Autodesk Fusion 360 part; units mm, degrees
note: some values were not read from the file. Chosen so that the rebuilt part matches the saved one: which bodies a step acts on.
(part 2 of 3)
extrude "Extrude1'''''''''''''''''''''''" add sketch "FingerTech_Mini_Switch_Envelope_Outline" along normal blind 6.35 from surface at 49 separate body makes body 27 in component "FingerTech_Mini_Switch_Envelope"
sketch "FingerTech_Mount_Holes_M2" plane through (0, 0, 0) normal (0, 0, 1) x (1, 0, 0) in component "FingerTech_Mini_Switch_Envelope"
  circle A0 centre (38.19, -70) radius 1
  circle A1 centre (45.81, -70) radius 1
extrude "Extrude2''''''''''''''''" cut sketch "FingerTech_Mount_Holes_M2" along normal blind 9 from surface at 48 bodies 27 in component "FingerTech_Mini_Switch_Envelope"
sketch "FingerTech_Access_Patch" plane through (0, 0, 0) normal (0, 0, 1) x (1, 0, 0) in component "Top_Cover"
  line L0 (31, -79) -> (53, -79)
  line L1 (53, -79) -> (53, -61)
  line L2 (53, -61) -> (31, -61)
  line L3 (31, -61) -> (31, -79)
extrude "Extrude7''''" add sketch "FingerTech_Access_Patch" along normal blind 2 from surface at 83 bodies 6 in component "Top_Cover"
sketch "FingerTech_Hex_Access_6mm" plane through (0, 0, 0) normal (0, 0, 1) x (1, 0, 0) in component "Top_Cover"
  circle A0 centre (42, -70) radius 3
extrude "Extrude8''" cut sketch "FingerTech_Hex_Access_6mm" along normal blind 4 from surface at 82 bodies 6 in component "Top_Cover"
sketch "Lifter_Spatula_62mm_Side_Profile" plane through (0, 0, 0) normal (1, 0, 0) x (0, 0, -1) in component "Lifter_Spatula_62mm"
  line L0 (-27, 70) -> (-5.8, 112)
  line L1 (-5.8, 112) -> (-8.5, 112)
  line L2 (-8.5, 112) -> (-30, 72)
  line L3 (-30, 72) -> (-27, 70)
extrude "Extrude1''''''''''''''''''''''''" add sketch "Lifter_Spatula_62mm_Side_Profile" along normal blind 62 from surface at -31 separate body makes body 28 in component "Lifter_Spatula_62mm"
sketch "Lifter_Hinge_Boss_Outline" plane through (0, 0, 0) normal (0, 0, 1) x (1, 0, 0) in component "Lifter_Hinge_Boss"
  line L0 (-30, 64) -> (30, 64)
  line L1 (30, 64) -> (30, 74)
  line L2 (30, 74) -> (-30, 74)
  line L3 (-30, 74) -> (-30, 64)
extrude "Extrude1'''''''''''''''''''''''''" add sketch "Lifter_Hinge_Boss_Outline" along normal blind 9 from surface at 27 separate body makes body 29 in component "Lifter_Hinge_Boss"
sketch "Hinge_Clearance_Bore_6p4mm" plane through (0, 0, 0) normal (1, 0, 0) x (0, 0, -1) in component "Lifter_Hinge_Boss"
  circle A0 centre (-31.5, 68) radius 3.2
extrude "Extrude2'''''''''''''''''" cut sketch "Hinge_Clearance_Bore_6p4mm" along normal mid plane 100 bodies 29 in component "Lifter_Hinge_Boss"
sketch "Lifter_Pivot_Support_L_Outline" plane through (0, 0, 0) normal (0, 0, 1) x (1, 0, 0) in component "Lifter_Pivot_Support_L"
  line L0 (-35, 61) -> (-32, 61)
  line L1 (-32, 61) -> (-32, 76)
  line L2 (-32, 76) -> (-35, 76)
  line L3 (-35, 76) -> (-35, 61)
extrude "Extrude1''''''''''''''''''''''''''" add sketch "Lifter_Pivot_Support_L_Outline" along normal blind 17 from surface at 24 separate body makes body 30 in component "Lifter_Pivot_Support_L"
sketch "Lifter_Pivot_Support_R_Outline" plane through (0, 0, 0) normal (0, 0, 1) x (1, 0, 0) in component "Lifter_Pivot_Support_R"
  line L0 (32, 61) -> (35, 61)
  line L1 (35, 61) -> (35, 76)
  line L2 (35, 76) -> (32, 76)
  line L3 (32, 76) -> (32, 61)
extrude "Extrude1'''''''''''''''''''''''''''" add sketch "Lifter_Pivot_Support_R_Outline" along normal blind 17 from surface at 24 separate body makes body 31 in component "Lifter_Pivot_Support_R"
sketch "Left_Pivot_Bore_6p4mm" plane through (0, 0, 0) normal (1, 0, 0) x (0, 0, -1) in component "Lifter_Pivot_Support_L"
  circle A0 centre (-31.5, 68) radius 3.2
extrude "Extrude2''''''''''''''''''" cut sketch "Left_Pivot_Bore_6p4mm" along normal mid plane 100 bodies 30 in component "Lifter_Pivot_Support_L"
sketch "Right_Pivot_Bore_6p4mm" plane through (0, 0, 0) normal (1, 0, 0) x (0, 0, -1) in component "Lifter_Pivot_Support_R"
  circle A0 centre (-31.5, 68) radius 3.2
extrude "Extrude2'''''''''''''''''''" cut sketch "Right_Pivot_Bore_6p4mm" along normal mid plane 100 bodies 31 in component "Lifter_Pivot_Support_R"
sketch "Lifter_Pivot_Pin_6mm_Section" plane through (0, 0, 0) normal (1, 0, 0) x (0, 0, -1) in component "Lifter_Pivot_Pin_6mm"
  circle A0 centre (-31.5, 68) radius 3
extrude "Extrude1''''''''''''''''''''''''''''" add sketch "Lifter_Pivot_Pin_6mm_Section" along normal blind 72 from surface at -36 separate body makes body 32 in component "Lifter_Pivot_Pin_6mm"
sketch "Pin_End_Trim_L" plane through (0, 0, 0) normal (1, 0, 0) x (0, 0, -1) in component "Lifter_Pivot_Pin_6mm"
  circle A0 centre (-31.5, 68) radius 3.5
extrude "Extrude2''''''''''''''''''''" cut sketch "Pin_End_Trim_L" along normal blind 1.3 from surface at -36.1 bodies 32 in component "Lifter_Pivot_Pin_6mm"
sketch "Pin_End_Trim_R" plane through (0, 0, 0) normal (1, 0, 0) x (0, 0, -1) in component "Lifter_Pivot_Pin_6mm"
  circle A0 centre (-31.5, 68) radius 3.5
extrude "Extrude3''''''''''''''''" cut sketch "Pin_End_Trim_R" along normal blind 1.3 from surface at 34.8 bodies 32 in component "Lifter_Pivot_Pin_6mm"
sketch "Load_Path_To_Base_L" plane through (0, 0, 0) normal (0, 0, 1) x (1, 0, 0) in component "Lifter_Pivot_Support_L"
  line L0 (-35, 61) -> (-25, 61)
  line L1 (-25, 61) -> (-25, 76)
  line L2 (-25, 76) -> (-35, 76)
  line L3 (-35, 76) -> (-35, 61)
extrude "Extrude3'''''''''''''''''" add sketch "Load_Path_To_Base_L" along normal blind 20 from surface at 5 bodies 30 in component "Lifter_Pivot_Support_L"
sketch "Lifter_Support_Base_M3_Clear_L" plane through (0, 0, 0) normal (0, 0, 1) x (1, 0, 0) in component "Base_Plate_Al"
  circle A0 centre (-29.5, 64.5) radius 1.7
  circle A1 centre (-29.5, 72.5) radius 1.7
extrude "Lifter_Support_Base_M3_Clear_L_Cut" cut sketch "Lifter_Support_Base_M3_Clear_L" along normal blind 2.2 from surface at 2.9 bodies 1 in component "Base_Plate_Al"
sketch "Lifter_Support_M3_Tap_L" plane through (0, 0, 0) normal (0, 0, 1) x (1, 0, 0) in component "Lifter_Pivot_Support_L"
  circle A0 centre (-29.5, 64.5) radius 1.25
  circle A1 centre (-29.5, 72.5) radius 1.25
extrude "Lifter_Support_M3_Tap_L_Cut" cut sketch "Lifter_Support_M3_Tap_L" along normal blind 8.1 from surface at 4.9 bodies 30 in component "Lifter_Pivot_Support_L"
sketch "Load_Path_To_Base_R" plane through (0, 0, 0) normal (0, 0, 1) x (1, 0, 0) in component "Lifter_Pivot_Support_R"
  line L0 (25, 61) -> (35, 61)
  line L1 (35, 61) -> (35, 76)
  line L2 (35, 76) -> (25, 76)
  line L3 (25, 76) -> (25, 61)
extrude "Extrude3''''''''''''''''''" add sketch "Load_Path_To_Base_R" along normal blind 20 from surface at 5 bodies 31 in component "Lifter_Pivot_Support_R"
sketch "Lifter_Support_Base_M3_Clear_R" plane through (0, 0, 0) normal (0, 0, 1) x (1, 0, 0) in component "Base_Plate_Al"
  circle A0 centre (29.5, 64.5) radius 1.7
  circle A1 centre (29.5, 72.5) radius 1.7
extrude "Lifter_Support_Base_M3_Clear_R_Cut" cut sketch "Lifter_Support_Base_M3_Clear_R" along normal blind 2.2 from surface at 2.9 bodies 1 in component "Base_Plate_Al"
sketch "Lifter_Support_M3_Tap_R" plane through (0, 0, 0) normal (0, 0, 1) x (1, 0, 0) in component "Lifter_Pivot_Support_R"
  circle A0 centre (29.5, 64.5) radius 1.25
  circle A1 centre (29.5, 72.5) radius 1.25
extrude "Lifter_Support_M3_Tap_R_Cut" cut sketch "Lifter_Support_M3_Tap_R" along normal blind 8.1 from surface at 4.9 bodies 31 in component "Lifter_Pivot_Support_R"
sketch "Repeat_40kg_Servo_MaxEnvelope_Outline" plane through (0, 0, 0) normal (0, 0, 1) x (1, 0, 0) in component "Repeat_40kg_Servo_MaxEnvelope"
  line L0 (-25.1, 12) -> (31.1, 12)
  line L1 (31.1, 12) -> (31.1, 56.5)
  line L2 (31.1, 56.5) -> (-25.1, 56.5)
  line L3 (-25.1, 56.5) -> (-25.1, 12)
extrude "Extrude1'''''''''''''''''''''''''''''" add sketch "Repeat_40kg_Servo_MaxEnvelope_Outline" along normal blind 20 from surface at 12 separate body makes body 33 in component "Repeat_40kg_Servo_MaxEnvelope"
sketch "Lifter_Servo_Base_Rail_L_Outline" plane through (0, 0, 0) normal (0, 0, 1) x (1, 0, 0) in component "Lifter_Servo_Base_Rail_L"
  line L0 (-25.1, 14) -> (-21.1, 14)
  line L1 (-21.1, 14) -> (-21.1, 54)
  line L2 (-21.1, 54) -> (-25.1, 54)
  line L3 (-25.1, 54) -> (-25.1, 14)
extrude "Extrude1''''''''''''''''''''''''''''''" add sketch "Lifter_Servo_Base_Rail_L_Outline" along normal blind 7 from surface at 5 separate body makes body 34 in component "Lifter_Servo_Base_Rail_L"
sketch "Lifter_Servo_Base_Rail_R_Outline" plane through (0, 0, 0) normal (0, 0, 1) x (1, 0, 0) in component "Lifter_Servo_Base_Rail_R"
  line L0 (27.1, 14) -> (31.1, 14)
  line L1 (31.1, 14) -> (31.1, 54)
  line L2 (31.1, 54) -> (27.1, 54)
  line L3 (27.1, 54) -> (27.1, 14)
extrude "Extrude1'''''''''''''''''''''''''''''''" add sketch "Lifter_Servo_Base_Rail_R_Outline" along normal blind 7 from surface at 5 separate body makes body 35 in component "Lifter_Servo_Base_Rail_R"
sketch "Lifter_Aluminium_Horn_Profile" plane through (0, 0, 0) normal (1, 0, 0) x (0, 0, -1) in component "Lifter_Aluminium_Horn"
  line L0 (-25, 38) -> (-25, 61)
  line L1 (-25, 61) -> (-19, 61)
  line L2 (-19, 61) -> (-19, 38)
  line L3 (-19, 38) -> (-25, 38)
extrude "Extrude1''''''''''''''''''''''''''''''''" add sketch "Lifter_Aluminium_Horn_Profile" along normal blind 3 from surface at -28.1 separate body makes body 36 in component "Lifter_Aluminium_Horn"
sketch "Lifter_Aluminium_Horn" plane through (0, 0, 0) normal (1, 0, 0) x (0, 0, -1) in component "Lifter_Aluminium_Horn"
  circle A0 centre (-22, 42) radius 1.6
  circle A1 centre (-22, 57) radius 1.6
extrude "Extrude2'''''''''''''''''''''" cut sketch "Lifter_Aluminium_Horn" along normal mid plane 100 bodies 36 in component "Lifter_Aluminium_Horn"
sketch "Lifter_Connecting_Rod_Profile" plane through (0, 0, 0) normal (1, 0, 0) x (0, 0, -1) in component "Lifter_Connecting_Rod"
  line L0 (-18.8868, 53.0875) -> (-49.6277, 61.1068)
  line L1 (-49.6277, 61.1068) -> (-48.1132, 66.9125)
  line L2 (-48.1132, 66.9125) -> (-17.3723, 58.8932)
  line L3 (-17.3723, 58.8932) -> (-18.8868, 53.0875)
extrude "Extrude1'''''''''''''''''''''''''''''''''" add sketch "Lifter_Connecting_Rod_Profile" along normal blind 3 from surface at -31.1 separate body makes body 37 in component "Lifter_Connecting_Rod"
sketch "Lifter_Connecting_Rod" plane through (0, 0, 0) normal (1, 0, 0) x (0, 0, -1) in component "Lifter_Connecting_Rod"
  circle A0 centre (-22, 57) radius 1.6
  circle A1 centre (-45, 63) radius 1.6
extrude "Extrude2''''''''''''''''''''''" cut sketch "Lifter_Connecting_Rod" along normal mid plane 100 bodies 37 in component "Lifter_Connecting_Rod"
sketch "Welded_Lifter_Lever" plane through (0, 0, 0) normal (0, 0, 1) x (1, 0, 0) in component "Lifter_Hinge_Boss"
  line L0 (-28.1, 59) -> (-25.1, 59)
  line L1 (-25.1, 59) -> (-25.1, 69)
  line L2 (-25.1, 69) -> (-28.1, 69)
  line L3 (-28.1, 69) -> (-28.1, 59)
extrude "Extrude3'''''''''''''''''''" add sketch "Welded_Lifter_Lever" along normal blind 18 from surface at 31 bodies 29 in component "Lifter_Hinge_Boss"
sketch "Lever_M3_Clevis_Hole" plane through (0, 0, 0) normal (1, 0, 0) x (0, 0, -1) in component "Lifter_Hinge_Boss"
  circle A0 centre (-45, 63) radius 1.6
extrude "Extrude4'''''''''''" cut sketch "Lever_M3_Clevis_Hole" along normal mid plane 100 bodies 29 in component "Lifter_Hinge_Boss"
sketch "Lifter_Lower_Hard_Stop_Outline" plane through (0, 0, 0) normal (0, 0, 1) x (1, 0, 0) in component "Lifter_Lower_Hard_Stop"
  line L0 (-10, 82) -> (10, 82)
  line L1 (10, 82) -> (10, 89)
  line L2 (10, 89) -> (-10, 89)
  line L3 (-10, 89) -> (-10, 82)
extrude "Extrude1''''''''''''''''''''''''''''''''''" add sketch "Lifter_Lower_Hard_Stop_Outline" along normal blind 8 from surface at 5 separate body makes body 38 in component "Lifter_Lower_Hard_Stop"
sketch "Servo_Output_Shaft_D3" plane through (0, 0, 0) normal (1, 0, 0) x (0, 0, -1) in component "Repeat_40kg_Servo_MaxEnvelope"
  circle A0 centre (-22, 42) radius 1.5
extrude "Extrude2'''''''''''''''''''''''" add sketch "Servo_Output_Shaft_D3" along normal blind 4 from surface at -28.1 bodies 33 in component "Repeat_40kg_Servo_MaxEnvelope"
sketch "Flange_Clearance_L" plane through (0, 0, 0) normal (0, 0, 1) x (1, 0, 0) in component "Lifter_Pivot_Support_L"
  line L0 (-32, 60.9) -> (-24.9, 60.9)
  line L1 (-24.9, 60.9) -> (-24.9, 76.1)
  line L2 (-24.9, 76.1) -> (-32, 76.1)
  line L3 (-32, 76.1) -> (-32, 60.9)
extrude "Extrude5'''''''" cut sketch "Flange_Clearance_L" along normal blind 11.1 from surface at 14 bodies 30 in component "Lifter_Pivot_Support_L"
sketch "Flange_Clearance_R" plane through (0, 0, 0) normal (0, 0, 1) x (1, 0, 0) in component "Lifter_Pivot_Support_R"
  line L0 (24.9, 60.9) -> (32, 60.9)
  line L1 (32, 60.9) -> (32, 76.1)
  line L2 (32, 76.1) -> (24.9, 76.1)
  line L3 (24.9, 76.1) -> (24.9, 60.9)
extrude "Extrude5''''''''" cut sketch "Flange_Clearance_R" along normal blind 11.1 from surface at 14 bodies 31 in component "Lifter_Pivot_Support_R"
sketch "Lever_Repair_Pivot_Bore" plane through (0, 0, 0) normal (1, 0, 0) x (0, 0, -1) in component "Lifter_Hinge_Boss"
  circle A0 centre (-31.5, 68) radius 3.2
extrude "Extrude5'''''''''" cut sketch "Lever_Repair_Pivot_Bore" along normal mid plane 100 bodies 29 in component "Lifter_Hinge_Boss"
sketch "BBB_22mm_Gearmotor_L_Section" plane through (0, 0, 0) normal (1, 0, 0) x (0, 0, -1) in component "BBB_22mm_Gearmotor_L"
  circle A0 centre (-21, 0) radius 11
extrude "Extrude1'''''''''''''''''''''''''''''''''''" add sketch "BBB_22mm_Gearmotor_L_Section" along normal blind 49 from surface at -58 separate body makes body 39 in component "BBB_22mm_Gearmotor_L"
sketch "BBB_4mm_Output_Shaft_L_Section" plane through (0, 0, 0) normal (1, 0, 0) x (0, 0, -1) in component "BBB_4mm_Output_Shaft_L"
  circle A0 centre (-21, 0) radius 2
extrude "Extrude1''''''''''''''''''''''''''''''''''''" add sketch "BBB_4mm_Output_Shaft_L_Section" along normal blind 14 from surface at -72 separate body makes body 40 in component "BBB_4mm_Output_Shaft_L"
sketch "BBB_Face_Mount_26mm_L_Outline" plane through (0, 0, 0) normal (0, 0, 1) x (1, 0, 0) in component "BBB_Face_Mount_26mm_L"
  line L0 (-61, -13) -> (-58, -13)
  line L1 (-58, -13) -> (-58, 13)
  line L2 (-58, 13) -> (-61, 13)
  line L3 (-61, 13) -> (-61, -13)
extrude "Extrude1'''''''''''''''''''''''''''''''''''''" add sketch "BBB_Face_Mount_26mm_L_Outline" along normal blind 26 from surface at 8 separate body makes body 41 in component "BBB_Face_Mount_26mm_L"
sketch "Face_Motor_Bore_L" plane through (0, 0, 0) normal (1, 0, 0) x (0, 0, -1) in component "BBB_Face_Mount_26mm_L"
  circle A0 centre (-21, 0) radius 11.1
extrude "Face_Motor_Bore_L_Cut" cut sketch "Face_Motor_Bore_L" along normal blind 3.2 from surface at -61.1 bodies 41 in component "BBB_Face_Mount_26mm_L"
sketch "Face_M3_20mm_Pattern_L" plane through (0, 0, 0) normal (1, 0, 0) x (0, 0, -1) in component "BBB_Face_Mount_26mm_L"
  circle A0 centre (-11, -10) radius 1.6
  circle A1 centre (-31, -10) radius 1.6
  circle A2 centre (-11, 10) radius 1.6
  circle A3 centre (-31, 10) radius 1.6
extrude "Face_M3_20mm_Pattern_L_Cut" cut sketch "Face_M3_20mm_Pattern_L" along normal blind 3.2 from surface at -61.1 bodies 41 in component "BBB_Face_Mount_26mm_L"
sketch "BBB_Motor_Cradle_L_Outline" plane through (0, 0, 0) normal (0, 0, 1) x (1, 0, 0) in component "BBB_Motor_Cradle_L"
  line L0 (-58, -20) -> (-48, -20)
  line L1 (-48, -20) -> (-48, 20)
  line L2 (-48, 20) -> (-58, 20)
  line L3 (-58, 20) -> (-58, -20)
extrude "Extrude1''''''''''''''''''''''''''''''''''''''" add sketch "BBB_Motor_Cradle_L_Outline" along normal blind 32 from surface at 5 separate body makes body 42 in component "BBB_Motor_Cradle_L"
sketch "Cradle_Motor_Bore_L" plane through (0, 0, 0) normal (1, 0, 0) x (0, 0, -1) in component "BBB_Motor_Cradle_L"
  circle A0 centre (-21, 0) radius 11.1
extrude "Cradle_Motor_Bore_L_Cut" cut sketch "Cradle_Motor_Bore_L" along normal blind 10.2 from surface at -58.1 bodies 42 in component "BBB_Motor_Cradle_L"
sketch "Cradle_M3_Face_Tap_L" plane through (0, 0, 0) normal (1, 0, 0) x (0, 0, -1) in component "BBB_Motor_Cradle_L"
  circle A0 centre (-11, -10) radius 1.25
  circle A1 centre (-31, -10) radius 1.25
  circle A2 centre (-11, 10) radius 1.25
  circle A3 centre (-31, 10) radius 1.25
extrude "Cradle_M3_Face_Tap_L_Cut" cut sketch "Cradle_M3_Face_Tap_L" along normal blind 10.2 from surface at -58.1 bodies 42 in component "BBB_Motor_Cradle_L"
sketch "Cradle_M3_Base_Tap_L" plane through (0, 0, 0) normal (0, 0, 1) x (1, 0, 0) in component "BBB_Motor_Cradle_L"
  circle A0 centre (-53, -16) radius 1.25
  circle A1 centre (-53, 16) radius 1.25
extrude "Cradle_M3_Base_Tap_L_Cut" cut sketch "Cradle_M3_Base_Tap_L" along normal blind 12.1 from surface at 4.9 bodies 42 in component "BBB_Motor_Cradle_L"
sketch "Cradle_M3_Base_Clear_L" plane through (0, 0, 0) normal (0, 0, 1) x (1, 0, 0) in component "Base_Plate_Al"
  circle A0 centre (-53, -16) radius 1.7
  circle A1 centre (-53, 16) radius 1.7
extrude "Cradle_M3_Base_Clear_L_Cut" cut sketch "Cradle_M3_Base_Clear_L" along normal blind 2.2 from surface at 2.9 bodies 1 in component "Base_Plate_Al"
sketch "Hub_16p2_Counterbore_L" plane through (0, 0, 0) normal (1, 0, 0) x (0, 0, -1) in component "Left_Wheel"
  circle A0 centre (-21, 0) radius 8.1
extrude "Hub_16p2_Counterbore_L_Cut" cut sketch "Hub_16p2_Counterbore_L" along normal blind 6.4 from surface at -67.2 bodies 4 in component "Left_Wheel"
sketch "Shaft_4p2_Blind_Bore_L" plane through (0, 0, 0) normal (1, 0, 0) x (0, 0, -1) in component "Left_Wheel"
  circle A0 centre (-21, 0) radius 2.1
extrude "Shaft_4p2_Blind_Bore_L_Cut" cut sketch "Shaft_4p2_Blind_Bore_L" along normal blind 5.1 from surface at -72.2 bodies 4 in component "Left_Wheel"
sketch "Wheel_M3_12p7_Pattern_L" plane through (0, 0, 0) normal (1, 0, 0) x (0, 0, -1) in component "Left_Wheel"
  circle A0 centre (-21, -6.35) radius 1.7
  circle A1 centre (-21, 6.35) radius 1.7
extrude "Wheel_M3_12p7_Pattern_L_Cut" cut sketch "Wheel_M3_12p7_Pattern_L" along normal blind 13 from surface at -80.1 bodies 4 in component "Left_Wheel"
sketch "Repeat_4mm_Clamp_Hub_L_Section" plane through (0, 0, 0) normal (1, 0, 0) x (0, 0, -1) in component "Repeat_4mm_Clamp_Hub_L"
  circle A0 centre (-21, 0) radius 8
extrude "Extrude1'''''''''''''''''''''''''''''''''''''''" add sketch "Repeat_4mm_Clamp_Hub_L_Section" along normal blind 6 from surface at -67 separate body makes body 43 in component "Repeat_4mm_Clamp_Hub_L"
sketch "Hub_4mm_Shaft_Bore_L" plane through (0, 0, 0) normal (1, 0, 0) x (0, 0, -1) in component "Repeat_4mm_Clamp_Hub_L"
  circle A0 centre (-21, 0) radius 2
extrude "Hub_4mm_Shaft_Bore_L_Cut" cut sketch "Hub_4mm_Shaft_Bore_L" along normal blind 6.2 from surface at -67.1 bodies 43 in component "Repeat_4mm_Clamp_Hub_L"
sketch "Hub_M3_12p7_Tap_L" plane through (0, 0, 0) normal (1, 0, 0) x (0, 0, -1) in component "Repeat_4mm_Clamp_Hub_L"
  circle A0 centre (-21, -6.35) radius 1.25
  circle A1 centre (-21, 6.35) radius 1.25
extrude "Hub_M3_12p7_Tap_L_Cut" cut sketch "Hub_M3_12p7_Tap_L" along normal blind 6.2 from surface at -67.1 bodies 43 in component "Repeat_4mm_Clamp_Hub_L"
sketch "BBB_22mm_Gearmotor_R_Section" plane through (0, 0, 0) normal (1, 0, 0) x (0, 0, -1) in component "BBB_22mm_Gearmotor_R"
  circle A0 centre (-21, 0) radius 11
extrude "Extrude1''''''''''''''''''''''''''''''''''''''''" add sketch "BBB_22mm_Gearmotor_R_Section" along normal blind 49 from surface at 9 separate body makes body 44 in component "BBB_22mm_Gearmotor_R"
sketch "BBB_4mm_Output_Shaft_R_Section" plane through (0, 0, 0) normal (1, 0, 0) x (0, 0, -1) in component "BBB_4mm_Output_Shaft_R"
  circle A0 centre (-21, 0) radius 2
extrude "Extrude1'''''''''''''''''''''''''''''''''''''''''" add sketch "BBB_4mm_Output_Shaft_R_Section" along normal blind 14 from surface at 58 separate body makes body 45 in component "BBB_4mm_Output_Shaft_R"
sketch "BBB_Face_Mount_26mm_R_Outline" plane through (0, 0, 0) normal (0, 0, 1) x (1, 0, 0) in component "BBB_Face_Mount_26mm_R"
  line L0 (58, -13) -> (61, -13)
  line L1 (61, -13) -> (61, 13)
  line L2 (61, 13) -> (58, 13)
  line L3 (58, 13) -> (58, -13)
extrude "Extrude1''''''''''''''''''''''''''''''''''''''''''" add sketch "BBB_Face_Mount_26mm_R_Outline" along normal blind 26 from surface at 8 separate body makes body 46 in component "BBB_Face_Mount_26mm_R"
sketch "Face_Motor_Bore_R" plane through (0, 0, 0) normal (1, 0, 0) x (0, 0, -1) in component "BBB_Face_Mount_26mm_R"
  circle A0 centre (-21, 0) radius 11.1
extrude "Face_Motor_Bore_R_Cut" cut sketch "Face_Motor_Bore_R" along normal blind 3.2 from surface at 57.9 bodies 46 in component "BBB_Face_Mount_26mm_R"
sketch "Face_M3_20mm_Pattern_R" plane through (0, 0, 0) normal (1, 0, 0) x (0, 0, -1) in component "BBB_Face_Mount_26mm_R"
  circle A0 centre (-11, -10) radius 1.6
  circle A1 centre (-31, -10) radius 1.6
  circle A2 centre (-11, 10) radius 1.6
  circle A3 centre (-31, 10) radius 1.6
extrude "Face_M3_20mm_Pattern_R_Cut" cut sketch "Face_M3_20mm_Pattern_R" along normal blind 3.2 from surface at 57.9 bodies 46 in component "BBB_Face_Mount_26mm_R"
sketch "BBB_Motor_Cradle_R_Outline" plane through (0, 0, 0) normal (0, 0, 1) x (1, 0, 0) in component "BBB_Motor_Cradle_R"
  line L0 (48, -20) -> (58, -20)
  line L1 (58, -20) -> (58, 20)
  line L2 (58, 20) -> (48, 20)
  line L3 (48, 20) -> (48, -20)
extrude "Extrude1'''''''''''''''''''''''''''''''''''''''''''" add sketch "BBB_Motor_Cradle_R_Outline" along normal blind 32 from surface at 5 separate body makes body 47 in component "BBB_Motor_Cradle_R"
sketch "Cradle_Motor_Bore_R" plane through (0, 0, 0) normal (1, 0, 0) x (0, 0, -1) in component "BBB_Motor_Cradle_R"
  circle A0 centre (-21, 0) radius 11.1
extrude "Cradle_Motor_Bore_R_Cut" cut sketch "Cradle_Motor_Bore_R" along normal blind 10.2 from surface at 47.9 bodies 47 in component "BBB_Motor_Cradle_R"
sketch "Cradle_M3_Face_Tap_R" plane through (0, 0, 0) normal (1, 0, 0) x (0, 0, -1) in component "BBB_Motor_Cradle_R"
  circle A0 centre (-11, -10) radius 1.25
  circle A1 centre (-31, -10) radius 1.25
  circle A2 centre (-11, 10) radius 1.25
  circle A3 centre (-31, 10) radius 1.25
extrude "Cradle_M3_Face_Tap_R_Cut" cut sketch "Cradle_M3_Face_Tap_R" along normal blind 10.2 from surface at 47.9 bodies 47 in component "BBB_Motor_Cradle_R"
sketch "Cradle_M3_Base_Tap_R" plane through (0, 0, 0) normal (0, 0, 1) x (1, 0, 0) in component "BBB_Motor_Cradle_R"
  circle A0 centre (53, -16) radius 1.25
  circle A1 centre (53, 16) radius 1.25
extrude "Cradle_M3_Base_Tap_R_Cut" cut sketch "Cradle_M3_Base_Tap_R" along normal blind 12.1 from surface at 4.9 bodies 47 in component "BBB_Motor_Cradle_R"
sketch "Cradle_M3_Base_Clear_R" plane through (0, 0, 0) normal (0, 0, 1) x (1, 0, 0) in component "Base_Plate_Al"
  circle A0 centre (53, -16) radius 1.7
  circle A1 centre (53, 16) radius 1.7
extrude "Cradle_M3_Base_Clear_R_Cut" cut sketch "Cradle_M3_Base_Clear_R" along normal blind 2.2 from surface at 2.9 bodies 1 in component "Base_Plate_Al"
sketch "Hub_16p2_Counterbore_R" plane through (0, 0, 0) normal (1, 0, 0) x (0, 0, -1) in component "Right_Wheel"
  circle A0 centre (-21, 0) radius 8.1
extrude "Hub_16p2_Counterbore_R_Cut" cut sketch "Hub_16p2_Counterbore_R" along normal blind 6.4 from surface at 60.8 bodies 5 in component "Right_Wheel"
sketch "Shaft_4p2_Blind_Bore_R" plane through (0, 0, 0) normal (1, 0, 0) x (0, 0, -1) in component "Right_Wheel"
  circle A0 centre (-21, 0) radius 2.1
extrude "Shaft_4p2_Blind_Bore_R_Cut" cut sketch "Shaft_4p2_Blind_Bore_R" along normal blind 5.1 from surface at 67.1 bodies 5 in component "Right_Wheel"
sketch "Wheel_M3_12p7_Pattern_R" plane through (0, 0, 0) normal (1, 0, 0) x (0, 0, -1) in component "Right_Wheel"
  circle A0 centre (-21, -6.35) radius 1.7
  circle A1 centre (-21, 6.35) radius 1.7
extrude "Wheel_M3_12p7_Pattern_R_Cut" cut sketch "Wheel_M3_12p7_Pattern_R" along normal blind 13 from surface at 67.1 bodies 5 in component "Right_Wheel"
sketch "Repeat_4mm_Clamp_Hub_R_Section" plane through (0, 0, 0) normal (1, 0, 0) x (0, 0, -1) in component "Repeat_4mm_Clamp_Hub_R"
  circle A0 centre (-21, 0) radius 8
extrude "Extrude1''''''''''''''''''''''''''''''''''''''''''''" add sketch "Repeat_4mm_Clamp_Hub_R_Section" along normal blind 6 from surface at 61 separate body makes body 48 in component "Repeat_4mm_Clamp_Hub_R"
sketch "Hub_4mm_Shaft_Bore_R" plane through (0, 0, 0) normal (1, 0, 0) x (0, 0, -1) in component "Repeat_4mm_Clamp_Hub_R"
  circle A0 centre (-21, 0) radius 2
extrude "Hub_4mm_Shaft_Bore_R_Cut" cut sketch "Hub_4mm_Shaft_Bore_R" along normal blind 6.2 from surface at 60.9 bodies 48 in component "Repeat_4mm_Clamp_Hub_R"
sketch "Hub_M3_12p7_Tap_R" plane through (0, 0, 0) normal (1, 0, 0) x (0, 0, -1) in component "Repeat_4mm_Clamp_Hub_R"
  circle A0 centre (-21, -6.35) radius 1.25
  circle A1 centre (-21, 6.35) radius 1.25
extrude "Hub_M3_12p7_Tap_R_Cut" cut sketch "Hub_M3_12p7_Tap_R" along normal blind 6.2 from surface at 60.9 bodies 48 in component "Repeat_4mm_Clamp_Hub_R"
sketch "BBB_Dual_Brushed_ESC_v2_Envelope_Outline" plane through (0, 0, 0) normal (0, 0, 1) x (1, 0, 0) in component "BBB_Dual_Brushed_ESC_v2_Envelope"
  line L0 (-8, -84) -> (12, -84)
  line L1 (12, -84) -> (12, -68)
  line L2 (12, -68) -> (-8, -68)
  line L3 (-8, -68) -> (-8, -84)
extrude "Extrude1'''''''''''''''''''''''''''''''''''''''''''''" add sketch "BBB_Dual_Brushed_ESC_v2_Envelope_Outline" along normal blind 5 from surface at 7 separate body makes body 49 in component "BBB_Dual_Brushed_ESC_v2_Envelope"
sketch "Battery_Tray_Rear_Clearance_L" plane through (0, 0, 0) normal (0, 0, 1) x (1, 0, 0) in component "BBB_Motor_Cradle_L"
  line L0 (-58.1, -20.1) -> (-47.9, -20.1)
  line L1 (-47.9, -20.1) -> (-47.9, -18)
  line L2 (-47.9, -18) -> (-58.1, -18)
  line L3 (-58.1, -18) -> (-58.1, -20.1)
extrude "Extrude5''''''''''" cut sketch "Battery_Tray_Rear_Clearance_L" along normal blind 7.1 from surface at 30 bodies 42 in component "BBB_Motor_Cradle_L"
sketch "Battery_Tray_Rear_Clearance_R" plane through (0, 0, 0) normal (0, 0, 1) x (1, 0, 0) in component "BBB_Motor_Cradle_R"
  line L0 (47.9, -20.1) -> (58.1, -20.1)
  line L1 (58.1, -20.1) -> (58.1, -18)
  line L2 (58.1, -18) -> (47.9, -18)
  line L3 (47.9, -18) -> (47.9, -20.1)
extrude "Extrude5'''''''''''" cut sketch "Battery_Tray_Rear_Clearance_R" along normal blind 7.1 from surface at 30 bodies 47 in component "BBB_Motor_Cradle_R"
sketch "Battery_Clamp_Bar_1_Outline" plane through (0, 0, 0) normal (0, 0, 1) x (1, 0, 0) in component "Battery_Clamp_Bar_1"
  line L0 (-78, -51) -> (78, -51)
  line L1 (78, -51) -> (78, -45)
  line L2 (78, -45) -> (-78, -45)
  line L3 (-78, -45) -> (-78, -51)
extrude "Extrude1''''''''''''''''''''''''''''''''''''''''''''''" add sketch "Battery_Clamp_Bar_1_Outline" along normal blind 6 from surface at 61.6 separate body makes body 50 in component "Battery_Clamp_Bar_1"
sketch "Clamp_M3_Tap_L_1" plane through (0, 0, 0) normal (1, 0, 0) x (0, 0, -1) in component "Battery_Clamp_Bar_1"
  circle A0 centre (-64.6, -48) radius 1.25
extrude "Extrude2''''''''''''''''''''''''" cut sketch "Clamp_M3_Tap_L_1" along normal blind 10.2 from surface at -78.1 bodies 50 in component "Battery_Clamp_Bar_1"
sketch "Clamp_M3_Tap_R_1" plane through (0, 0, 0) normal (1, 0, 0) x (0, 0, -1) in component "Battery_Clamp_Bar_1"
  circle A0 centre (-64.6, -48) radius 1.25
extrude "Extrude3''''''''''''''''''''" cut sketch "Clamp_M3_Tap_R_1" along normal blind 10.2 from surface at 67.9 bodies 50 in component "Battery_Clamp_Bar_1"
sketch "Clamp_M3_Clear_L_1" plane through (0, 0, 0) normal (1, 0, 0) x (0, 0, -1) in component "Left_Side_Plate_Al"
  circle A0 centre (-64.6, -48) radius 1.7
extrude "Extrude8'''" cut sketch "Clamp_M3_Clear_L_1" along normal blind 2.2 from surface at -80.1 bodies 2 in component "Left_Side_Plate_Al"
sketch "Clamp_M3_Clear_R_1" plane through (0, 0, 0) normal (1, 0, 0) x (0, 0, -1) in component "Right_Side_Plate_Al"
  circle A0 centre (-64.6, -48) radius 1.7
extrude "Extrude8''''" cut sketch "Clamp_M3_Clear_R_1" along normal blind 2.2 from surface at 77.9 bodies 3 in component "Right_Side_Plate_Al"
sketch "Battery_Clamp_Bar_2_Outline" plane through (0, 0, 0) normal (0, 0, 1) x (1, 0, 0) in component "Battery_Clamp_Bar_2"
  line L0 (-78, -31) -> (78, -31)
  line L1 (78, -31) -> (78, -25)
  line L2 (78, -25) -> (-78, -25)
  line L3 (-78, -25) -> (-78, -31)
extrude "Extrude1'''''''''''''''''''''''''''''''''''''''''''''''" add sketch "Battery_Clamp_Bar_2_Outline" along normal blind 6 from surface at 61.6 separate body makes body 51 in component "Battery_Clamp_Bar_2"
sketch "Clamp_M3_Tap_L_2" plane through (0, 0, 0) normal (1, 0, 0) x (0, 0, -1) in component "Battery_Clamp_Bar_2"
  circle A0 centre (-64.6, -28) radius 1.25
extrude "Extrude2'''''''''''''''''''''''''" cut sketch "Clamp_M3_Tap_L_2" along normal blind 10.2 from surface at -78.1 bodies 51 in component "Battery_Clamp_Bar_2"
sketch "Clamp_M3_Tap_R_2" plane through (0, 0, 0) normal (1, 0, 0) x (0, 0, -1) in component "Battery_Clamp_Bar_2"
  circle A0 centre (-64.6, -28) radius 1.25
extrude "Extrude3'''''''''''''''''''''" cut sketch "Clamp_M3_Tap_R_2" along normal blind 10.2 from surface at 67.9 bodies 51 in component "Battery_Clamp_Bar_2"
sketch "Clamp_M3_Clear_L_2" plane through (0, 0, 0) normal (1, 0, 0) x (0, 0, -1) in component "Left_Side_Plate_Al"
  circle A0 centre (-64.6, -28) radius 1.7
extrude "Extrude9'" cut sketch "Clamp_M3_Clear_L_2" along normal blind 2.2 from surface at -80.1 bodies 2 in component "Left_Side_Plate_Al"
sketch "Clamp_M3_Clear_R_2" plane through (0, 0, 0) normal (1, 0, 0) x (0, 0, -1) in component "Right_Side_Plate_Al"
  circle A0 centre (-64.6, -28) radius 1.7
extrude "Extrude9''" cut sketch "Clamp_M3_Clear_R_2" along normal blind 2.2 from surface at 77.9 bodies 3 in component "Right_Side_Plate_Al"
sketch "Lifter_Servo_Clamp_Bar_L_Outline" plane through (0, 0, 0) normal (0, 0, 1) x (1, 0, 0) in component "Lifter_Servo_Clamp_Bar_L"
  line L0 (-15, -15) -> (-9, -15)
  line L1 (-9, -15) -> (-9, 60)
  line L2 (-9, 60) -> (-15, 60)
  line L3 (-15, 60) -> (-15, -15)
extrude "Extrude1''''''''''''''''''''''''''''''''''''''''''''''''" add sketch "Lifter_Servo_Clamp_Bar_L_Outline" along normal blind 2 from surface at 32 separate body makes body 52 in component "Lifter_Servo_Clamp_Bar_L"
sketch "Clamp_Bar_M3_Clear_L" plane through (0, 0, 0) normal (0, 0, 1) x (1, 0, 0) in component "Lifter_Servo_Clamp_Bar_L"
  circle A0 centre (-12, -15) radius 1.7
  circle A1 centre (-12, 60) radius 1.7
extrude "Extrude2''''''''''''''''''''''''''" cut sketch "Clamp_Bar_M3_Clear_L" along normal blind 2.2 from surface at 31.9 bodies 52 in component "Lifter_Servo_Clamp_Bar_L"
sketch "Lifter_Servo_Clamp_Post_L_Rear_Outline" plane through (0, 0, 0) normal (0, 0, 1) x (1, 0, 0) in component "Lifter_Servo_Clamp_Post_L_Rear"
  line L0 (-15, -18) -> (-9, -18)
  line L1 (-9, -18) -> (-9, -12)
  line L2 (-9, -12) -> (-15, -12)
  line L3 (-15, -12) -> (-15, -18)
extrude "Extrude1'''''''''''''''''''''''''''''''''''''''''''''''''" add sketch "Lifter_Servo_Clamp_Post_L_Rear_Outline" along normal blind 27 from surface at 5 separate body makes body 53 in component "Lifter_Servo_Clamp_Post_L_Rear"
sketch "Clamp_Post_M3_Tap_L_Rear" plane through (0, 0, 0) normal (0, 0, 1) x (1, 0, 0) in component "Lifter_Servo_Clamp_Post_L_Rear"
  circle A0 centre (-12, -15) radius 1.25
extrude "Extrude2'''''''''''''''''''''''''''" cut sketch "Clamp_Post_M3_Tap_L_Rear" along normal blind 27.2 from surface at 4.9 bodies 53 in component "Lifter_Servo_Clamp_Post_L_Rear"
sketch "Lifter_Servo_Clamp_Post_L_Front_Outline" plane through (0, 0, 0) normal (0, 0, 1) x (1, 0, 0) in component "Lifter_Servo_Clamp_Post_L_Front"
  line L0 (-15, 57) -> (-9, 57)
  line L1 (-9, 57) -> (-9, 63)
  line L2 (-9, 63) -> (-15, 63)
  line L3 (-15, 63) -> (-15, 57)
extrude "Extrude1''''''''''''''''''''''''''''''''''''''''''''''''''" add sketch "Lifter_Servo_Clamp_Post_L_Front_Outline" along normal blind 27 from surface at 5 separate body makes body 54 in component "Lifter_Servo_Clamp_Post_L_Front"
sketch "Clamp_Post_M3_Tap_L_Front" plane through (0, 0, 0) normal (0, 0, 1) x (1, 0, 0) in component "Lifter_Servo_Clamp_Post_L_Front"
  circle A0 centre (-12, 60) radius 1.25
extrude "Extrude2''''''''''''''''''''''''''''" cut sketch "Clamp_Post_M3_Tap_L_Front" along normal blind 27.2 from surface at 4.9 bodies 54 in component "Lifter_Servo_Clamp_Post_L_Front"
sketch "Lifter_Servo_Clamp_Bar_R_Outline" plane through (0, 0, 0) normal (0, 0, 1) x (1, 0, 0) in component "Lifter_Servo_Clamp_Bar_R"
  line L0 (9, -15) -> (15, -15)
  line L1 (15, -15) -> (15, 60)
  line L2 (15, 60) -> (9, 60)
  line L3 (9, 60) -> (9, -15)
extrude "Extrude1'''''''''''''''''''''''''''''''''''''''''''''''''''" add sketch "Lifter_Servo_Clamp_Bar_R_Outline" along normal blind 2 from surface at 32 separate body makes body 55 in component "Lifter_Servo_Clamp_Bar_R"
sketch "Clamp_Bar_M3_Clear_R" plane through (0, 0, 0) normal (0, 0, 1) x (1, 0, 0) in component "Lifter_Servo_Clamp_Bar_R"
  circle A0 centre (12, -15) radius 1.7
  circle A1 centre (12, 60) radius 1.7
extrude "Extrude2'''''''''''''''''''''''''''''" cut sketch "Clamp_Bar_M3_Clear_R" along normal blind 2.2 from surface at 31.9 bodies 55 in component "Lifter_Servo_Clamp_Bar_R"
sketch "Lifter_Servo_Clamp_Post_R_Rear_Outline" plane through (0, 0, 0) normal (0, 0, 1) x (1, 0, 0) in component "Lifter_Servo_Clamp_Post_R_Rear"
  line L0 (9, -18) -> (15, -18)
  line L1 (15, -18) -> (15, -12)
  line L2 (15, -12) -> (9, -12)
  line L3 (9, -12) -> (9, -18)
extrude "Extrude1''''''''''''''''''''''''''''''''''''''''''''''''''''" add sketch "Lifter_Servo_Clamp_Post_R_Rear_Outline" along normal blind 27 from surface at 5 separate body makes body 56 in component "Lifter_Servo_Clamp_Post_R_Rear"
sketch "Clamp_Post_M3_Tap_R_Rear" plane through (0, 0, 0) normal (0, 0, 1) x (1, 0, 0) in component "Lifter_Servo_Clamp_Post_R_Rear"
  circle A0 centre (12, -15) radius 1.25
extrude "Extrude2''''''''''''''''''''''''''''''" cut sketch "Clamp_Post_M3_Tap_R_Rear" along normal blind 27.2 from surface at 4.9 bodies 56 in component "Lifter_Servo_Clamp_Post_R_Rear"
sketch "Lifter_Servo_Clamp_Post_R_Front_Outline" plane through (0, 0, 0) normal (0, 0, 1) x (1, 0, 0) in component "Lifter_Servo_Clamp_Post_R_Front"
  line L0 (9, 57) -> (15, 57)
  line L1 (15, 57) -> (15, 63)
  line L2 (15, 63) -> (9, 63)
  line L3 (9, 63) -> (9, 57)
extrude "Extrude1'''''''''''''''''''''''''''''''''''''''''''''''''''''" add sketch "Lifter_Servo_Clamp_Post_R_Front_Outline" along normal blind 27 from surface at 5 separate body makes body 57 in component "Lifter_Servo_Clamp_Post_R_Front"
sketch "Clamp_Post_M3_Tap_R_Front" plane through (0, 0, 0) normal (0, 0, 1) x (1, 0, 0) in component "Lifter_Servo_Clamp_Post_R_Front"
  circle A0 centre (12, 60) radius 1.25
extrude "Extrude2'''''''''''''''''''''''''''''''" cut sketch "Clamp_Post_M3_Tap_R_Front" along normal blind 27.2 from surface at 4.9 bodies 57 in component "Lifter_Servo_Clamp_Post_R_Front"
sketch "Lifter_Servo_Clamp_Base_M3_Clear" plane through (0, 0, 0) normal (0, 0, 1) x (1, 0, 0) in component "Base_Plate_Al"
  circle A0 centre (-12, -15) radius 1.7
  circle A1 centre (-12, 60) radius 1.7
  circle A2 centre (12, -15) radius 1.7
  circle A3 centre (12, 60) radius 1.7
extrude "Extrude33" cut sketch "Lifter_Servo_Clamp_Base_M3_Clear" along normal blind 2.2 from surface at 2.9 bodies 1 in component "Base_Plate_Al"
sketch "Pin_Clip_Groove_L" plane through (0, 0, 0) normal (1, 0, 0) x (0, 0, -1) in component "Lifter_Pivot_Pin_6mm"
  circle A0 centre (-31.5, 68) radius 3.05
  circle A1 centre (-31.5, 68) radius 2.5
extrude "Extrude4''''''''''''" cut sketch "Pin_Clip_Groove_L" along normal blind 0.8 from surface at -31.4 bodies 32 in component "Lifter_Pivot_Pin_6mm"
sketch "Pin_Clip_Groove_R" plane through (0, 0, 0) normal (1, 0, 0) x (0, 0, -1) in component "Lifter_Pivot_Pin_6mm"
  circle A0 centre (-31.5, 68) radius 3.05
  circle A1 centre (-31.5, 68) radius 2.5
extrude "Extrude5''''''''''''" cut sketch "Pin_Clip_Groove_R" along normal blind 0.8 from surface at 30.6 bodies 32 in component "Lifter_Pivot_Pin_6mm"
sketch "C_Clip_Section_L" plane through (0, 0, 0) normal (1, 0, 0) x (0, 0, -1) in component "Lifter_Pin_C_Clip_L"
  circle A0 centre (-31.5, 68) radius 5
  circle A1 centre (-31.5, 68) radius 2.5
extrude "Extrude1''''''''''''''''''''''''''''''''''''''''''''''''''''''" add sketch "C_Clip_Section_L" along normal blind 0.8 from surface at -31.4 separate body makes body 58 in component "Lifter_Pin_C_Clip_L"
sketch "C_Clip_Opening_L" plane through (0, 0, 0) normal (1, 0, 0) x (0, 0, -1) in component "Lifter_Pin_C_Clip_L"
  line L0 (-30.4, 70.2) -> (-32.6, 70.2)
  line L1 (-32.6, 70.2) -> (-32.6, 73.2)
  line L2 (-32.6, 73.2) -> (-30.4, 73.2)
  line L3 (-30.4, 73.2) -> (-30.4, 70.2)
extrude "Extrude2''''''''''''''''''''''''''''''''" cut sketch "C_Clip_Opening_L" along normal blind 1 from surface at -31.5 bodies 58 in component "Lifter_Pin_C_Clip_L"
sketch "C_Clip_Section_R" plane through (0, 0, 0) normal (1, 0, 0) x (0, 0, -1) in component "Lifter_Pin_C_Clip_R"
  circle A0 centre (-31.5, 68) radius 5
  circle A1 centre (-31.5, 68) radius 2.5
extrude "Extrude1'''''''''''''''''''''''''''''''''''''''''''''''''''''''" add sketch "C_Clip_Section_R" along normal blind 0.8 from surface at 30.6 separate body makes body 59 in component "Lifter_Pin_C_Clip_R"
sketch "C_Clip_Opening_R" plane through (0, 0, 0) normal (1, 0, 0) x (0, 0, -1) in component "Lifter_Pin_C_Clip_R"
  line L0 (-30.4, 70.2) -> (-32.6, 70.2)
  line L1 (-32.6, 70.2) -> (-32.6, 73.2)
  line L2 (-32.6, 73.2) -> (-30.4, 73.2)
  line L3 (-30.4, 73.2) -> (-30.4, 70.2)
extrude "Extrude2'''''''''''''''''''''''''''''''''" cut sketch "C_Clip_Opening_R" along normal blind 1 from surface at 30.5 bodies 59 in component "Lifter_Pin_C_Clip_R"
sketch "C_Clip_OD_8p4_L" plane through (0, 0, 0) normal (1, 0, 0) x (0, 0, -1) in component "Lifter_Pin_C_Clip_L"
  circle A0 centre (-31.5, 68) radius 5.1
  circle A1 centre (-31.5, 68) radius 4.2
extrude "Extrude3''''''''''''''''''''''" cut sketch "C_Clip_OD_8p4_L" along normal blind 1 from surface at -31.5 bodies 58 in component "Lifter_Pin_C_Clip_L"
sketch "C_Clip_OD_8p4_R" plane through (0, 0, 0) normal (1, 0, 0) x (0, 0, -1) in component "Lifter_Pin_C_Clip_R"
  circle A0 centre (-31.5, 68) radius 5.1
  circle A1 centre (-31.5, 68) radius 4.2
extrude "Extrude3'''''''''''''''''''''''" cut sketch "C_Clip_OD_8p4_R" along normal blind 1 from surface at 30.5 bodies 59 in component "Lifter_Pin_C_Clip_R"
sketch "C_Clip_OD_8p0_L" plane through (0, 0, 0) normal (1, 0, 0) x (0, 0, -1) in component "Lifter_Pin_C_Clip_L"
  circle A0 centre (-31.5, 68) radius 5.1
  circle A1 centre (-31.5, 68) radius 4
extrude "Extrude4'''''''''''''" cut sketch "C_Clip_OD_8p0_L" along normal blind 1 from surface at -31.5 bodies 58 in component "Lifter_Pin_C_Clip_L"
sketch "C_Clip_OD_8p0_R" plane through (0, 0, 0) normal (1, 0, 0) x (0, 0, -1) in component "Lifter_Pin_C_Clip_R"
  circle A0 centre (-31.5, 68) radius 5.1
  circle A1 centre (-31.5, 68) radius 4
extrude "Extrude4''''''''''''''" cut sketch "C_Clip_OD_8p0_R" along normal blind 1 from surface at 30.5 bodies 59 in component "Lifter_Pin_C_Clip_R"
ref_plane "WorkPlane1" through (0, 0, 0) normal (1, 0, 0) x (0, 1, 0) in component "Lifter_Lower_Hard_Stop"
sketch "Lower_Stop_Raised_To_Blade_Profile" plane through (0, 0, 0) normal (1, 0, 0) x (0, 0, -1) in component "Lifter_Lower_Hard_Stop"
  line L0 (-12, 82) -> (-12, 89)
  line L1 (-12, 89) -> (-17.4095, 89)
  line L2 (-17.4095, 89) -> (-20.9429, 82)
  line L3 (-20.9429, 82) -> (-12, 82)
extrude "Lower_Stop_Raised_To_Blade" add sketch "Lower_Stop_Raised_To_Blade_Profile" along normal mid plane 20 bodies 38 in component "Lifter_Lower_Hard_Stop"
ref_plane "WorkPlane1" through (24, 0, 0) normal (1, 0, 0) x (0, 1, 0) in component "Lifter_Pivot_Support_R"
sketch "Lifter_Upper_Stop_45deg_Profile" plane through (24, 0, 0) normal (1, 0, 0) x (0, 0, -1) in component "Lifter_Pivot_Support_R"
  line L0 (-36.5, 63.5) -> (-36.5, 66.636)
  line L1 (-36.5, 66.636) -> (-38.9246, 69.0607)
  line L2 (-38.9246, 69.0607) -> (-39.5, 72)
  line L3 (-39.5, 72) -> (-46, 72)
  line L4 (-46, 72) -> (-46, 63.5)
  line L5 (-46, 63.5) -> (-36.5, 63.5)
extrude "Lifter_Upper_Stop_45deg" add sketch "Lifter_Upper_Stop_45deg_Profile" along normal mid plane 16 separate body makes body 60 in component "Lifter_Pivot_Support_R"
component "01_Chassis" placed x (1, 0, 0) y (0, 1, 0) z (0, 0, 1) at (0, 0, 0)
component "02_Drivetrain" placed x (1, 0, 0) y (0, 1, 0) z (0, 0, 1) at (0, 0, 0)
component "05_Electronics" placed x (1, 0, 0) y (0, 1, 0) z (0, 0, 1) at (0, 0, 0)
component "06_3D_Printed" placed x (1, 0, 0) y (0, 1, 0) z (0, 0, 1) at (0, 0, 0)
component "07_Wedge_Lifter_Option" placed x (1, 0, 0) y (0, 1, 0) z (0, 0, 1) at (0, 0, 0)
component "09_3S_Drive_Upgrade" placed x (1, 0, 0) y (0, 1, 0) z (0, 0, 1) at (0, 0, 0)
component "10_Battery_Restraints" placed x (1, 0, 0) y (0, 1, 0) z (0, 0, 1) at (0, 0, 0)
component "Base_Plate_Al" placed x (1, 0, 0) y (0, 1, 0) z (0, 0, 1) at (0, 0, 0) in component "01_Chassis"
component "Left_Side_Plate_Al" placed x (1, 0, 0) y (0, 1, 0) z (0, 0, 1) at (0, 0, 0) in component "01_Chassis"
component "Right_Side_Plate_Al" placed x (1, 0, 0) y (0, 1, 0) z (0, 0, 1) at (0, 0, 0) in component "01_Chassis"
component "Top_Cover" placed x (1, 0, 0) y (0, 1, 0) z (0, 0, 1) at (0, 0, 0) in component "01_Chassis"
component "Front_Wedge_L" placed x (1, 0, 0) y (0, 1, 0) z (0, 0, 1) at (0, 0, 0) in component "01_Chassis"
component "Front_Wedge_R" placed x (1, 0, 0) y (0, 1, 0) z (0, 0, 1) at (0, 0, 0) in component "01_Chassis"
component "Standoffs_Fasteners" placed x (1, 0, 0) y (0, 1, 0) z (0, 0, 1) at (0, 0, 0) in component "01_Chassis"
component "Left_Wheel" placed x (1, 0, 0) y (0, 1, 0) z (0, 0, 1) at (0, 0, 0) in component "02_Drivetrain"
component "Right_Wheel" placed x (1, 0, 0) y (0, 1, 0) z (0, 0, 1) at (0, 0, 0) in component "02_Drivetrain"
component "Battery_and_Tray" placed x (1, 0, 0) y (0, 1, 0) z (0, 0, 1) at (0, 0, 0) in component "05_Electronics"
component "Rx_ER6" placed x (1, 0, 0) y (0, 1, 0) z (0, 0, 1) at (0, 0, 0) in component "05_Electronics"
component "UBEC_5A" placed x (1, 0, 0) y (0, 1, 0) z (0, 0, 1) at (0, 0, 0) in component "05_Electronics"
component "FingerTech_Mini_Switch_Envelope" placed x (1, 0, 0) y (0, 1, 0) z (0, 0, 1) at (0, 0, 0) in component "05_Electronics"
component "BBB_Dual_Brushed_ESC_v2_Envelope" placed x (1, 0, 0) y (0, 1, 0) z (0, 0, 1) at (0, 0, 0) in component "05_Electronics"
component "Wire_Clips" placed x (1, 0, 0) y (0, 1, 0) z (0, 0, 1) at (0, 0, 0) in component "06_3D_Printed"
component "Non_Structural_Covers" placed x (1, 0, 0) y (0, 1, 0) z (0, 0, 1) at (0, 0, 0) in component "06_3D_Printed"
component "TPU_Bumpers" placed x (1, 0, 0) y (0, 1, 0) z (0, 0, 1) at (0, 0, 0) in component "06_3D_Printed"
component "Battery_Holder" placed x (1, 0, 0) y (0, 1, 0) z (0, 0, 1) at (0, 0, 0) in component "06_3D_Printed"
component "Batt_Post_1" placed x (1, 0, 0) y (0, 1, 0) z (0, 0, 1) at (0, 0, 0) in component "06_3D_Printed"
component "Batt_Post_2" placed x (1, 0, 0) y (0, 1, 0) z (0, 0, 1) at (0, 0, 0) in component "06_3D_Printed"
component "Batt_Post_3" placed x (1, 0, 0) y (0, 1, 0) z (0, 0, 1) at (0, 0, 0) in component "06_3D_Printed"
component "Batt_Post_4" placed x (1, 0, 0) y (0, 1, 0) z (0, 0, 1) at (0, 0, 0) in component "06_3D_Printed"
component "Disconnect_Post_1" placed x (1, 0, 0) y (0, 1, 0) z (0, 0, 1) at (0, 0, 0) in component "06_3D_Printed"
component "Disconnect_Post_2" placed x (1, 0, 0) y (0, 1, 0) z (0, 0, 1) at (0, 0, 0) in component "06_3D_Printed"
component "Holder_Rx_ER6" placed x (1, 0, 0) y (0, 1, 0) z (0, 0, 1) at (0, 0, 0) in component "06_3D_Printed"
component "Holder_UBEC_5A" placed x (1, 0, 0) y (0, 1, 0) z (0, 0, 1) at (0, 0, 0) in component "06_3D_Printed"
component "FingerTech_Switch_Adapter" placed x (1, 0, 0) y (0, 1, 0) z (0, 0, 1) at (0, 0, 0) in component "06_3D_Printed"
component "Rear_Panel" placed x (1, 0, 0) y (0, 1, 0) z (0, 0, 1) at (0, 0, 0) in component "Non_Structural_Covers"
component "06_3D_Printed" placed x (1, 0, 0) y (0, 1, 0) z (0, 0, 1) at (0, 0, 0) in component "TPU_Bumpers"
component "Lifter_Spatula_62mm" placed x (1, 0, 0) y (0, 1, 0) z (0, 0, 1) at (0, 0, 0) in component "07_Wedge_Lifter_Option"
component "Lifter_Hinge_Boss" placed x (1, 0, 0) y (0, 1, 0) z (0, 0, 1) at (0, 0, 0) in component "07_Wedge_Lifter_Option"
component "Lifter_Pivot_Support_L" placed x (1, 0, 0) y (0, 1, 0) z (0, 0, 1) at (0, 0, 0) in component "07_Wedge_Lifter_Option"
component "Lifter_Pivot_Support_R" placed x (1, 0, 0) y (0, 1, 0) z (0, 0, 1) at (0, 0, 0) in component "07_Wedge_Lifter_Option"
component "Lifter_Pivot_Pin_6mm" placed x (1, 0, 0) y (0, 1, 0) z (0, 0, 1) at (0, 0, 0) in component "07_Wedge_Lifter_Option"
component "Repeat_40kg_Servo_MaxEnvelope" placed x (1, 0, 0) y (0, 1, 0) z (0, 0, 1) at (0, 0, 0) in component "07_Wedge_Lifter_Option"
component "Lifter_Servo_Base_Rail_L" placed x (1, 0, 0) y (0, 1, 0) z (0, 0, 1) at (0, 0, 0) in component "07_Wedge_Lifter_Option"
component "Lifter_Servo_Base_Rail_R" placed x (1, 0, 0) y (0, 1, 0) z (0, 0, 1) at (0, 0, 0) in component "07_Wedge_Lifter_Option"
component "Lifter_Aluminium_Horn" placed x (1, 0, 0) y (0, 1, 0) z (0, 0, 1) at (0, 0, 0) in component "07_Wedge_Lifter_Option"
component "Lifter_Connecting_Rod" placed x (1, 0, 0) y (0, 1, 0) z (0, 0, 1) at (0, 0, 0) in component "07_Wedge_Lifter_Option"
component "Lifter_Lower_Hard_Stop" placed x (1, 0, 0) y (0, 1, 0) z (0, 0, 1) at (0, 0, 0) in component "07_Wedge_Lifter_Option"
component "Lifter_Servo_Clamp_Bar_L" placed x (1, 0, 0) y (0, 1, 0) z (0, 0, 1) at (0, 0, 0) in component "07_Wedge_Lifter_Option"
component "Lifter_Servo_Clamp_Post_L_Rear" placed x (1, 0, 0) y (0, 1, 0) z (0, 0, 1) at (0, 0, 0) in component "07_Wedge_Lifter_Option"
component "Lifter_Servo_Clamp_Post_L_Front" placed x (1, 0, 0) y (0, 1, 0) z (0, 0, 1) at (0, 0, 0) in component "07_Wedge_Lifter_Option"
component "Lifter_Servo_Clamp_Bar_R" placed x (1, 0, 0) y (0, 1, 0) z (0, 0, 1) at (0, 0, 0) in component "07_Wedge_Lifter_Option"
component "Lifter_Servo_Clamp_Post_R_Rear" placed x (1, 0, 0) y (0, 1, 0) z (0, 0, 1) at (0, 0, 0) in component "07_Wedge_Lifter_Option"
component "Lifter_Servo_Clamp_Post_R_Front" placed x (1, 0, 0) y (0, 1, 0) z (0, 0, 1) at (0, 0, 0) in component "07_Wedge_Lifter_Option"
component "Lifter_Pin_C_Clip_L" placed x (1, 0, 0) y (0, 1, 0) z (0, 0, 1) at (0, 0, 0) in component "07_Wedge_Lifter_Option"
component "Lifter_Pin_C_Clip_R" placed x (1, 0, 0) y (0, 1, 0) z (0, 0, 1) at (0, 0, 0) in component "07_Wedge_Lifter_Option"
component "BBB_22mm_Gearmotor_L" placed x (1, 0, 0) y (0, 1, 0) z (0, 0, 1) at (0, 0, 0) in component "09_3S_Drive_Upgrade"
component "BBB_4mm_Output_Shaft_L" placed x (1, 0, 0) y (0, 1, 0) z (0, 0, 1) at (0, 0, 0) in component "09_3S_Drive_Upgrade"
component "BBB_Face_Mount_26mm_L" placed x (1, 0, 0) y (0, 1, 0) z (0, 0, 1) at (0, 0, 0) in component "09_3S_Drive_Upgrade"
component "BBB_Motor_Cradle_L" placed x (1, 0, 0) y (0, 1, 0) z (0, 0, 1) at (0, 0, 0) in component "09_3S_Drive_Upgrade"
component "Repeat_4mm_Clamp_Hub_L" placed x (1, 0, 0) y (0, 1, 0) z (0, 0, 1) at (0, 0, 0) in component "09_3S_Drive_Upgrade"
component "BBB_22mm_Gearmotor_R" placed x (1, 0, 0) y (0, 1, 0) z (0, 0, 1) at (0, 0, 0) in component "09_3S_Drive_Upgrade"
component "BBB_4mm_Output_Shaft_R" placed x (1, 0, 0) y (0, 1, 0) z (0, 0, 1) at (0, 0, 0) in component "09_3S_Drive_Upgrade"
component "BBB_Face_Mount_26mm_R" placed x (1, 0, 0) y (0, 1, 0) z (0, 0, 1) at (0, 0, 0) in component "09_3S_Drive_Upgrade"
component "BBB_Motor_Cradle_R" placed x (1, 0, 0) y (0, 1, 0) z (0, 0, 1) at (0, 0, 0) in component "09_3S_Drive_Upgrade"
component "Repeat_4mm_Clamp_Hub_R" placed x (1, 0, 0) y (0, 1, 0) z (0, 0, 1) at (0, 0, 0) in component "09_3S_Drive_Upgrade"
component "Battery_Clamp_Bar_1" placed x (1, 0, 0) y (0, 1, 0) z (0, 0, 1) at (0, 0, 0) in component "10_Battery_Restraints"
component "Battery_Clamp_Bar_2" placed x (1, 0, 0) y (0, 1, 0) z (0, 0, 1) at (0, 0, 0) in component "10_Battery_Restraints"
equation "body_L = 180 mm" comment "Body length"
equation "body_W = 160 mm" comment "Body width incl. wheels"
equation "body_H = 80 mm" comment "Chassis height - raised from 70mm to give spinner sweep safe clearance under top cover"
equation "base_t = 2 mm" comment "DECIDED 2026-09-23: 2 mm aluminium plate (user approved)"
equation "side_t = 2 mm" comment "DECIDED 2026-09-23: 2 mm aluminium plate (user approved)"
equation "ground_clearance = 3 mm" comment "Ground clearance target"
equation "wheel_OD = 42 mm" comment "CONFIRMED: 42mm TT-motor wheel"
equation "wheel_W = 19 mm" comment "CONFIRMED (typical TT wheel width; verify against actual supplier spec)"
equation "motor_OD = 25 mm" comment "Gear motor housing envelope"
equation "pcb_L = 60 mm" comment "Control PCB placeholder length"
equation "pcb_W = 50 mm" comment "Control PCB placeholder width"
equation "pcb_keepout_H = 22 mm" comment "PCB top keepout height (placeholder)"
equation "assembly_clearance = 1 mm" comment "Generic assembly clearance"
equation "d14 = body_W"
equation "d15 = body_L"
equation "d16 = wheel_W"
equation "d17 = wheel_OD"
equation "d18 = wheel_W"
equation "d19 = wheel_OD"
equation "d20 = pcb_W"
equation "d21 = pcb_L"
equation "d26 = body_W"
equation "d27 = body_L"
equation "d28 = -base_t"
equation "d56 = -body_W / 2"
equation "d58 = body_H - base_t"
equation "d59 = body_L"
equation "d60 = side_t"